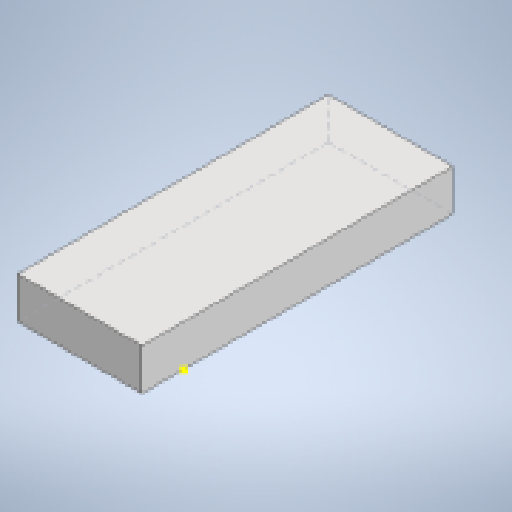
# Autodesk Inventor part: FlexK7V2
Saved by Autodesk Inventor 2023 (Build 270158000, 158)
## iProperties
Created: 2023-03-29
Part Number: FlexK7V2
Material: Generic
Document SubType Name: Modeling
Designer: Nathann
Density: 1 g/cm^3
Appearance: Default
Author: Nathann
Autodesk Inventor part; units mm, degrees
ref_plane "YZ Plane" through (0, 0, 0) normal (1, 0, 0) x (0, 1, 0)
ref_plane "XZ Plane" through (0, 0, 0) normal (0, 1, 0) x (-1, 0, 0)
ref_plane "XY Plane" through (0, 0, 0) normal (0, 0, 1) x (1, 0, 0)
sketch "Sketch1" plane through (0, 0, 0) normal (0, 1, 0) x (-1, 0, 0)
  line L0 (0, 0) -> (100, 0)
  line L1 (100, 0) -> (100, -150)
  line L2 (100, -150) -> (0, -150)
  line L3 (0, -150) -> (0, 0)
  line L4 (0, 0) -> (20, 0)
  line L5 (20, 0) -> (20, -150)
  line L6 (20, -150) -> (0, -150)
  line L7 (0, -150) -> (0, 0)
  line L8 (100, 0) -> (80, 0)
  line L9 (80, 0) -> (80, -150)
  line L10 (80, -150) -> (100, -150)
  line L11 (100, -150) -> (100, 0)
  dimension "d0" = 100
  dimension "d1" = 150
  dimension "d2" = 20
  dimension "d3" = 20
  dimension "d4" = 150
  dimension "d5" = 150
  constraints: 24 end point, 6 parallel, 3 horizontal, 3 perpendicular, 1 point on line
  measures "d0" distance of L0.start L0.end
  measures "d1" distance of L2.end L0.start
  measures "d2" distance of L9.end L10.end
  measures "d3" distance of L5.end L6.end
  measures "d4" distance of L4.end L5.end
  measures "d5" distance of L8.end L9.end
extrude "Extrusion1" add sketch "Sketch1" along normal blind 20 contours L0 L9 L2 L5
sketch "Sketch2" plane through (0, 20, 0) normal (0, 1, 0) x (1, 0, 0)
  point P0 (0, 0)
body "Solid1"
